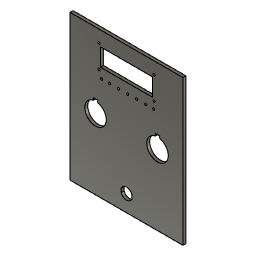
lazy-welder-chassis (Autodesk Fusion 360 design; units mm, degrees)
Autodesk Fusion 360 part; units mm, degrees
sketch "Sketch1" plane through (0, 0, 0) normal (0, 1, 0) x (1, 0, 0)
  line L0 (0, 0) -> (0, -197.9)
  line L1 (0, -197.9) -> (153.8, -197.9)
  line L2 (153.8, -197.9) -> (153.8, 0)
  line L3 (153.8, 0) -> (0, 0)
  line L4 (41.45, -177.9) -> (112.35, -177.9)
  line L5 (112.35, -177.9) -> (112.35, -153.9)
  line L6 (112.35, -153.9) -> (41.45, -153.9)
  line L7 (41.45, -153.9) -> (41.45, -177.9)
  circle A0 centre (39.4, -181.4) radius 1.5
  circle A1 centre (102.95, -140.7) radius 1.5
  circle A2 centre (113.95, -140.7) radius 1.5
  circle A3 centre (90.65, -140.7) radius 1.5
  circle A4 centre (78.35, -140.7) radius 1.5
  circle A5 centre (66.05, -140.7) radius 1.5
  circle A6 centre (53.75, -140.7) radius 1.5
  circle A7 centre (42.75, -140.7) radius 1.5
  circle A8 centre (114.4, -181.4) radius 1.5
  line L8 (31.8, -113.1111) -> (37.6, -113.1111)
  line L9 (31.8, -113.1111) -> (31.8, -110.1111)
  line L10 (37.6, -113.1111) -> (37.6, -110.1111)
  arc A9 (37.6, -110.1111) -> (31.8, -110.1111) centre (34.7, -95.7) ccw
  line L11 (116.2, -113.1111) -> (122, -113.1111)
  line L12 (116.2, -113.1111) -> (116.2, -110.1111)
  line L13 (122, -113.1111) -> (122, -110.1111)
  arc A10 (122, -110.1111) -> (116.2, -110.1111) centre (119.1, -95.7) ccw
  circle A11 centre (114.4, -150.4) radius 1.5
  circle A12 centre (39.4, -150.4) radius 1.5
  line L14 (69.55, -25.0076) -> (69.55, -20.0924)
  line L15 (84.25, -25.0076) -> (84.25, -20.0924)
  arc A13 (69.55, -25.0076) -> (84.25, -25.0076) centre (76.9, -22.55) ccw
  arc A14 (84.25, -20.0924) -> (69.55, -20.0924) centre (76.9, -22.55) ccw
  point P0 (106.0012, -102.3717)
  point P1 (41.7115, -182.3254)
  dimension "d1" = 197.9
  dimension "d6" = 70.9
  dimension "d13" = 153.8
  dimension "d22" = 29.4
  dimension "d27" = 95.7
  dimension "d28" = 34.7
  dimension "d29" = 84.4
  dimension "d30" = 95.7
  dimension "d31" = 34.7
  dimension "d32" = 22.55
  dimension "d33" = 76.9
  dimension "d34" = 20
  dimension "d35" = 41.45
  dimension "d38" = 3
  dimension "d39" = 13.2
  dimension "d40" = 9.4
  dimension "d41" = 3
  dimension "d42" = 11
  dimension "d43" = 13.2
  dimension "d44" = 3
  dimension "d45" = 3
  dimension "d46" = 12.3
  dimension "d47" = 12.3
  dimension "d49" = 12.3
  dimension "d50" = 3
  dimension "d51" = 12.3
  dimension "d52" = 3
  dimension "d53" = 11
  dimension "d54" = 13.2
  dimension "d55" = 13.2
  dimension "d56" = 13.2
  dimension "d57" = 13.2
  dimension "d58" = 3
  dimension "d59" = 13.2
  dimension "d60" = 3
  dimension "d61" = 75
  dimension "d69" = 5.8
  dimension "d70" = 3
  dimension "d71" = 3
  dimension "d72" = 5.8
  dimension "d73" = 3
  dimension "d74" = 3
  dimension "d77" = 3
  dimension "d78" = 3
  dimension "d80" = 31
  dimension "d81" = 31
  dimension "d82" = 24
  dimension "d83" = 3.5
  dimension "d86" = 75
  dimension "d87" = 2.05
  dimension "d89" = 3
  dimension "d94" = 14.7
  dimension "d101" = 14.7
  dimension "d102" = 7.75
  constraint coincident L0.start L3.end
  constraint vertical L0
  constraint perpendicular L0 L1
  constraint perpendicular L1 L2
  constraint perpendicular L0 L3
  constraint horizontal L4
  constraint vertical L5
  constraint horizontal L6
  constraint vertical L7
  constraint coincident P0 A10
  constraint horizontal L8
  constraint perpendicular L8 L9
  constraint perpendicular L8 L10
  constraint horizontal L11
  constraint perpendicular L11 L12
  constraint perpendicular L11 L13
  constraint vertical L14
  constraint coincident L15.end A13
  constraint vertical L15
  constraint concentric A13 A14
  measures "d1" distance of L0.start L0.end
  measures "d6" distance of L4.start L4.end
  measures "d13" distance of L0.end L1.end
  measures "d22" diameter of A9
  measures "d27" distance of L3 A9.centre
  measures "d28" distance of L0 A9.centre
  measures "d29" horizontal distance of A10.centre A9.centre
  measures "d30" distance of L3 A10.centre
  measures "d31" distance of L2 A10.centre
  measures "d32" distance of L3 A13.centre
  measures "d33" distance of L0 A13.centre
  measures "d34" distance of L1 L4
  measures "d35" distance of L0 L7
  measures "d38" diameter of A1
  measures "d39" distance of L6 A1.centre
  measures "d40" distance of L5 A1.centre
  measures "d41" diameter of A2
  measures "d42" horizontal distance of A1.centre A2.centre
  measures "d43" distance of L6 A2.centre
  measures "d44" diameter of A3
  measures "d45" diameter of A4
  measures "d46" horizontal distance of A1.centre A3.centre
  measures "d47" horizontal distance of A3.centre A4.centre
  measures "d49" horizontal distance of A4.centre A5.centre
  measures "d50" diameter of A6
  measures "d51" horizontal distance of A5.centre A6.centre
  measures "d52" diameter of A7
  measures "d53" distance of A6.centre A7.centre
  measures "d54" distance of L6 A3.centre
  measures "d55" distance of L6 A4.centre
  measures "d56" distance of L6 A5.centre
  measures "d57" distance of L6 A6.centre
  measures "d58" diameter of A5
  measures "d59" distance of L6 A7.centre
  measures "d60" diameter of A8
  measures "d61" horizontal distance of A0.centre A8.centre
  measures "d69" distance of L8.start L8.end
  measures "d70" distance of L8.start L9.end
  measures "d71" distance of L8.end L10.end
  measures "d72" distance of L11.start L11.end
  measures "d73" distance of L11.start L12.end
  measures "d74" distance of L11.end L13.end
  measures "d77" diameter of A11
  measures "d78" diameter of A12
  measures "d80" vertical distance of A8.centre A11.centre
  measures "d81" vertical distance of A0.centre A12.centre
  measures "d82" distance of L4.start L6.end
  measures "d83" distance of L4 A0.centre
  measures "d86" distance of A11.centre A12.centre
  measures "d87" distance of L7 A0.centre
  measures "d89" diameter of A0
  measures "d94" radius of A10
  measures "d101" distance of L14 L15
  measures "d102" radius of A13
extrude "Extrude1" add sketch "Sketch1" along normal blind 4
